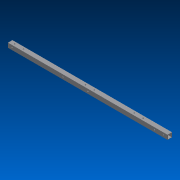
# Autodesk Inventor part: Bottom_Bar
Saved by Autodesk Inventor 2013 (Build 170138000, 138)
## iProperties
Created: 2013-07-13
Part Number: Bottom_Bar
Material: Aluminum 6061
Document SubType Name: Modeling
Designer: orange
Density: 1 g/cm^3
Author: orange
Autodesk Inventor part; units mm, degrees
ref_plane "YZ Plane" through (0, 0, 0) normal (1, 0, 0) x (0, 1, 0)
ref_plane "XZ Plane" through (0, 0, 0) normal (0, 1, 0) x (-1, 0, 0)
ref_plane "XY Plane" through (0, 0, 0) normal (0, 0, 1) x (1, 0, 0)
sketch "Sketch1" plane through (0, 0, 0) normal (1, 0, 0) x (0, 1, 0)
  line L0 (0, 0) -> (25.4, 0)
  line L1 (25.4, 0) -> (25.4, 25.4)
  line L2 (25.4, 25.4) -> (0, 25.4)
  line L3 (0, 25.4) -> (0, 0)
  line L4 (1.651, 1.651) -> (23.749, 1.651)
  line L5 (23.749, 1.651) -> (23.749, 23.749)
  line L6 (23.749, 23.749) -> (1.651, 23.749)
  line L7 (1.651, 23.749) -> (1.651, 1.651)
  dimension "d0" = 25.4
  dimension "d2" = 25.4
  dimension "d3" = 1.651
  dimension "d4" = 1.651
  dimension "d5" = 1.651
  dimension "d6" = 1.651
  constraints: 16 end point, 4 parallel, 2 horizontal, 2 perpendicular
  measures "d0" distance of L1.end L2.end
  measures "d2" distance of L2.end L0.start
  measures "d3" distance between parallel lines of L3 L7
  measures "d4" distance between parallel lines of L0 L4
  measures "d5" distance between parallel lines of L5 L1
  measures "d6" distance between parallel lines of L6 L2
extrude "Extrusion1" add sketch "Sketch1" along normal blind 914.4
sketch "Sketch3" plane through (0, 0, 0) normal (0, 0, -1) x (-1, 0, 0)
  line L0 (0, 25.4) -> (-914.4, 25.4) projected
  line L1 (-914.4, 0) -> (-914.4, 25.4) projected
  line L2 (0, 0) -> (-914.4, 0) projected
  point P0 (-889, 12.7)
  point P1 (-838.2, 12.7)
  dimension "d9" = 12.7
  dimension "d10" = 25.4
  dimension "d11" = 12.7
  dimension "d12" = 50.8
  measures "d9" distance from line of point (-889, 12.7) L0
  measures "d10" distance from line of point (-889, 12.7) L1
  measures "d11" distance from line of L2 point (-838.2, 12.7)
  measures "d12" distance of point (-889, 12.7) point (-838.2, 12.7)
hole "Hole1" at (889, 12.7, 0) at (838.2, 12.7, 0) direction (0, 0, 1) diameter 6.35 end through all
sketch "Sketch4" plane through (0, 25.4, 25.4) normal (0, 1, 0) x (1, 0, 0)
  line L0 (0, 0) -> (914.4, 0) projected
  line L1 (914.4, 25.4) -> (914.4, 0) projected
  line L2 (0, 25.4) -> (914.4, 25.4) projected
  line L3 (736.6, 25.4) -> (736.6, 0)
  point P0 (711.2, 12.7)
  point P1 (762, 12.7)
  dimension "d21" = 50.8
  dimension "d23" = 12.7
  dimension "d24" = 12.7
  dimension "d25" = 177.8
  dimension "d26" = 25.4
  constraints: 2 end point, 2 point on line, 1 perpendicular
  measures "d21" distance of point (762, 12.7) point (711.2, 12.7)
  measures "d23" distance from line of point (711.2, 12.7) L2
  measures "d24" distance from line of point (762, 12.7) L2
  measures "d25" distance between parallel lines of L3 L1
  measures "d26" distance from line of L3 point (711.2, 12.7)
hole "Hole2" at (711.2, 25.4, 12.7) at (762, 25.4, 12.7) direction (0, -1, 0) diameter 6.35 end through all
sketch "Sketch5" plane through (0, 0, 0) normal (0, 0, -1) x (-1, 0, 0)
  line L0 (0, 0) -> (0, 25.4) projected
  line L1 (0, 0) -> (-914.4, 0) projected
  point P0 (-314.7314, 12.7)
  point P1 (-22.6314, 12.7)
  dimension "d34" = 12.7
  dimension "d35" = 292.1
  dimension "d36" = 22.6314
  measures "d34" distance from line of L1 point (-22.631, 12.7)
  measures "d35" distance of point (-314.731, 12.7) point (-22.631, 12.7)
  measures "d36" distance from line of L0 point (-22.631, 12.7)
hole "Hole3" at (314.7314, 12.7, 0) at (22.6314, 12.7, 0) direction (0, 0, 1) diameter 6.35 end through all
sketch "Sketch6" plane through (0, 0, 0) normal (0, -1, 0) x (1, 0, 0)
  line L0 (0, 0) -> (914.4, 0) projected
  line L1 (914.4, 25.4) -> (914.4, 0) projected
  line L2 (0, 25.4) -> (914.4, 25.4) projected
  point P0 (431.8, 12.7)
  point P1 (482.6, 12.7)
  dimension "d44" = 50.8
  dimension "d46" = 12.7
  dimension "d47" = 12.7
  dimension "d48" = 431.8
  measures "d44" distance of point (431.8, 12.7) point (482.6, 12.7)
  measures "d46" distance from line of point (482.6, 12.7) L0
  measures "d47" distance from line of L2 point (431.8, 12.7)
  measures "d48" distance from line of point (482.6, 12.7) L1
hole "Hole4" at (431.8, 0, 12.7) at (482.6, 0, 12.7) direction (0, 1, 0) diameter 6.35 end through all
sketch "Sketch7" plane through (0, 0, 25.4) normal (0, 0, 1) x (1, 0, 0)
  line L0 (914.4, 25.4) -> (914.4, 0) projected
  line L1 (0, 25.4) -> (914.4, 25.4) projected
  point P0 (457.2, 12.7)
  dimension "d56" = 12.7
  dimension "d57" = 457.2
  measures "d56" distance from line of point (457.2, 12.7) L1
  measures "d57" distance from line of L0 point (457.2, 12.7)
hole "Hole5" at (457.2, 12.7, 25.4) direction (0, 0, -1) diameter 6.35 end through all
sketch "Sketch8" plane through (0, 0, 0) normal (0, -1, 0) x (1, 0, 0)
  line L0 (0, 25.4) -> (0, 0) projected
  point P0 (25.4, 12.7)
  point P1 (76.2, 12.7)
  dimension "d65" = 25.4
  dimension "d66" = 50.8
  measures "d65" distance from line of L0 point (25.4, 12.7)
  measures "d66" distance of point (76.2, 12.7) point (25.4, 12.7)
hole "Hole6" at (25.4, 0, 12.7) at (76.2, 0, 12.7) direction (0, 1, 0) diameter 6.35 end through all
body "Solid1"
